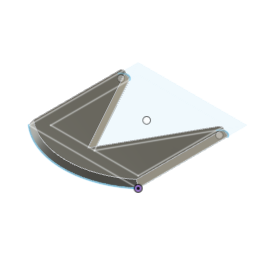
_JakeBreaker.9cdeba8a-3dd1-4735-84c7-f3c3d59873a5 (Autodesk Fusion 360 design; units mm, degrees)
Autodesk Fusion 360 part; units mm, degrees
sketch "Sketch1" plane through (0, 0, 0) normal (0, 0, 1) x (1, 0, 0)
  line L0 (0, 0) -> (-63.5, 0)
  line L1 (-63.5, 0) -> (-63.5, 63.5)
  line L2 (-63.5, 63.5) -> (0, 63.5)
  line L3 (0, 63.5) -> (0, 0)
  line L4 (-6.35, 6.35) -> (-57.15, 6.35)
  line L5 (-57.15, 6.35) -> (-57.15, 57.15)
  line L6 (-57.15, 57.15) -> (-6.35, 57.15)
  line L7 (-6.35, 57.15) -> (-6.35, 6.35)
  line L8 (-63.5, 63.5) -> (-31.75, 6.35)
  line L9 (0, 63.5) -> (-31.75, 6.35)
  arc A0 (-63.5, 0) -> (0, 0) centre (-31.75, 36.6899) ccw
  arc A1 (-57.15, 52.07) -> (-63.5, 52.07) centre (-60.325, 50.3061) ccw
  arc A2 (0, 52.07) -> (-6.35, 52.07) centre (-3.175, 50.3061) ccw
  dimension "d1" = 63.5
  dimension "d2" = 63.5
  dimension "d3" = 6.35
  constraint horizontal L0
  constraint vertical L1
  constraint horizontal L2
  constraint vertical L3
  constraint coincident L0.start L3.end
  constraint midpoint L4 L8.end
  constraint tangent L8 A1
  constraint coincident L1 A1.end
  constraint coincident L8 A1.start
  constraint coincident L5 A1.start
  constraint tangent L9 A2
  constraint coincident L3 A2.start
  constraint coincident L7 A2.end
  constraint coincident L9 A2.end
  measures "d1" distance of L0.start L0.end
  measures "d2" distance of L0.start L2.end
extrude "Extrude1" add sketch "Sketch1" along normal blind 3.175 draft -30 contours L0 A0 | L0 L1 L3 L4 L5 L7 A1 A2 | L4 L7 L9 | L4 L5 L8
